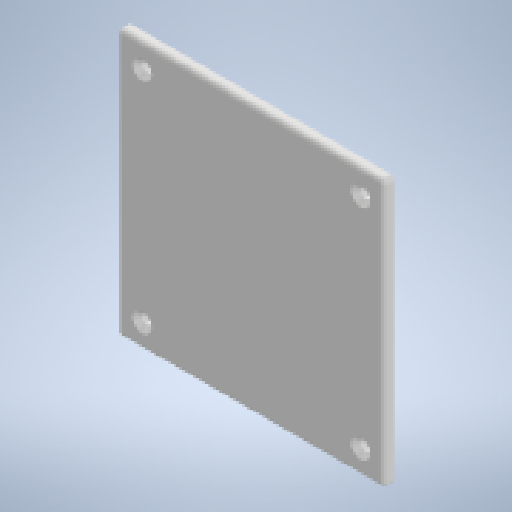
# Autodesk Inventor part: Lid
Saved by Autodesk Inventor 2024 (Build 280153000, 153)
## iProperties
Created: 2023-05-04
Part Number: Lid
Material: Generic
Document SubType Name: Modeling
Designer: cocqu
Density: 1 g/cm^3
Appearance: Default
Author: cocqu
Autodesk Inventor part; units mm, degrees
ref_plane "YZ Plane" through (0, 0, 0) normal (1, 0, 0) x (0, 1, 0)
ref_plane "XZ Plane" through (0, 0, 0) normal (0, 1, 0) x (-1, 0, 0)
ref_plane "XY Plane" through (0, 0, 0) normal (0, 0, 1) x (1, 0, 0)
sketch "Sketch2" plane through (0, 0, 0) normal (0, 0, 1) x (1, 0, 0)
  line L0 (-55, -55) -> (55, -55)
  line L1 (55, -55) -> (55, 55)
  line L2 (55, 55) -> (-55, 55)
  line L3 (-55, 55) -> (-55, -55)
  line L4 (-55, -55) -> (55, 55) construction
  line L5 (55, -55) -> (-55, 55) construction
  point P0 (0, 0)
  dimension "Lid_Width" = 110
  dimension "Lid_Length" = 110
  constraints: 12 end point, 2 midpoint, 2 parallel, 1 horizontal, 1 perpendicular
  measures "Lid_Width" distance of L2.end L1.end
  measures "Lid_Length" distance of L0.end L1.end
extrude "Extrusion1" add sketch "Sketch2" along normal blind 4
fillet "Fillet1" radius 2 8 edges at (-55, -55, 2) (-55, 55, 2) (55, 55, 2) (55, -55, 2) (55, 0, 4) (0, 55, 4) (-55, 0, 4) (0, -55, 4)
sketch "Sketch6" plane through (0, 0, 4) normal (0, 0, 1) x (1, 0, 0)
  circle A0 centre (-45, 45) radius 2
  line L0 (53, 55) -> (-53, 55) projected
  line L1 (-55, 53) -> (-55, -53) projected
  line L2 (0, 0) -> (0, 55) construction
  line L3 (0, 0) -> (-55, 0) construction
  circle A1 centre (45, 45) radius 2
  circle A2 centre (-45, -45) radius 2
  circle A3 centre (45, -45) radius 2
  dimension "d26" = 4
  dimension "d27" = 10
  dimension "d28" = 10
  constraints: 4 centre point, 4 end point, 3 symmetric about line, 2 midpoint, 3 other
  measures "d26" diameter of A0
  measures "d27" distance from line of L0 A0.centre
  measures "d28" distance from line of L1 A0.centre
extrude "Extrusion4" cut sketch "Sketch6" against normal blind 4
chamfer "Chamfer2" distance 2 angle 45 4 edges at (-47, 45, 4) (43, 45, 4) (43, -45, 4) (-47, -45, 4)
equation "\"Lid_Width\" = PCB_Width + 2 * Offset"
equation "\"Lid_Length\" = PCB_Length + 2 * Offset"
equation "\"d2\" = 2 * Wall_Thickness"
equation "\"d4\" = Wall_Thickness"
equation "\"d29\" = 2 * Wall_Thickness"
equation "\"d31\" = Wall_Thickness"
equation "\"Offset\" = 15"
equation "\"Wall_Thickness\" = 2"
equation "\"PCB_Width\" = 80"
equation "\"PCB_Length\" = 80"
body "Solid1"
